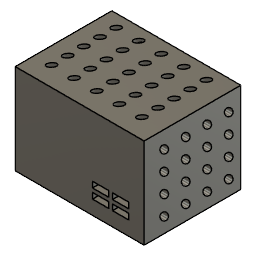
dronebox (Autodesk Fusion 360 design; units mm, degrees)
part number: 2026-05-27-13-25-45-977
Autodesk Fusion 360 part; units mm, degrees
sketch "Sketch12" plane through (0, 0, 0) normal (0, 0, 1) x (1, 0, 0)
  line L0 (50, 35) -> (-50, 35)
  line L1 (-50, 35) -> (-50, -35)
  line L2 (-50, -35) -> (50, -35)
  line L3 (50, -35) -> (50, 35)
  line L4 (50, 35) -> (-50, -35) construction
  line L5 (-50, 35) -> (50, -35) construction
  line L6 (-50, 35) -> (-50, 31)
  circle A0 centre (-20, 31) radius 1.6
  circle A1 centre (20, 31) radius 1.6
  circle A2 centre (-20, -31) radius 1.6
  circle A3 centre (20, -31) radius 1.6
  line L7 (42.5, -27.5) -> (42.5, 27.5)
  line L8 (42.5, 27.5) -> (-42.5, 27.5)
  line L9 (-42.5, 27.5) -> (-42.5, -27.5)
  line L10 (-42.5, -27.5) -> (42.5, -27.5)
  dimension "d61" = 100
  dimension "d62" = 70
  dimension "d63" = 4
  dimension "d64" = 30
  dimension "d65" = 3.2
  dimension "d66" = -7.5
  constraint horizontal L0
  constraint perpendicular L0 L1
  constraint parallel L0 L2
  constraint parallel L1 L3
  constraint coincident L4 origin
  constraint coincident L5 origin
  constraint perpendicular L0 L6
  measures "d61" distance of L1.end L2.end
  measures "d62" distance of L0.end L1.end
  measures "d63" distance of L0.end L6.end
  measures "d64" distance of L6.end A0.centre
  measures "d65" diameter of A0
extrude "Extrude12" add sketch "Sketch12" along normal blind 70 contours L0 L1 L2 L3 L6 | A0 | A1 | A2 | A3
extrude "Extrude13" cut sketch "Sketch12" along normal blind 15 contours A0 | A1 | A2 | A3
sketch "Sketch15" plane through (42.5, 0, 0) normal (-1, 0, 0) x (0, 0, 1)
  line L0 (0, 27.5) -> (0, -27.5)
  line L1 (0, -27.5) -> (70, -27.5)
  line L2 (70, -27.5) -> (70, 27.5)
  line L3 (70, 27.5) -> (0, 27.5)
sketch "Sketch16" plane through (-50, 0, 0) normal (-1, 0, 0) x (0, 0, 1)
  line L0 (0, 35) -> (0, -35)
  line L1 (0, -35) -> (70, -35)
  line L2 (70, -35) -> (70, 35)
  line L3 (70, 35) -> (0, 35)
  ellipse E0 centre (59.4117, -23.4278) end of major axis (56.6555, -26.4903) minor radius 2.5302
  line L4 (62.168, -20.3654) -> (56.6555, -26.4903) construction
  line L5 (57.5311, -21.7352) -> (61.2924, -25.1204) construction
  ellipse E1 centre (42.7451, -23.4278) end of major axis (39.9889, -26.4903) minor radius 2.5302
  ellipse E2 centre (26.0784, -23.4278) end of major axis (23.3222, -26.4903) minor radius 2.5302
  ellipse E3 centre (9.4117, -23.4278) end of major axis (6.6555, -26.4903) minor radius 2.5302
  ellipse E4 centre (59.4117, -8.4278) end of major axis (56.6555, -11.4903) minor radius 2.5302
  ellipse E5 centre (42.7451, -8.4278) end of major axis (39.9889, -11.4903) minor radius 2.5302
  ellipse E6 centre (26.0784, -8.4278) end of major axis (23.3222, -11.4903) minor radius 2.5302
  ellipse E7 centre (9.4117, -8.4278) end of major axis (6.6555, -11.4903) minor radius 2.5302
  ellipse E8 centre (59.4117, 6.5722) end of major axis (56.6555, 3.5097) minor radius 2.5302
  ellipse E9 centre (42.7451, 6.5722) end of major axis (39.9889, 3.5097) minor radius 2.5302
  ellipse E10 centre (26.0784, 6.5722) end of major axis (23.3222, 3.5097) minor radius 2.5302
  ellipse E11 centre (9.4117, 6.5722) end of major axis (6.6555, 3.5097) minor radius 2.5302
  ellipse E12 centre (59.4117, 21.5722) end of major axis (56.6555, 18.5097) minor radius 2.5302
  ellipse E13 centre (42.7451, 21.5722) end of major axis (39.9889, 18.5097) minor radius 2.5302
  ellipse E14 centre (26.0784, 21.5722) end of major axis (23.3222, 18.5097) minor radius 2.5302
  ellipse E15 centre (9.4117, 21.5722) end of major axis (6.6555, 18.5097) minor radius 2.5302
  dimension "d79" = -50
  dimension "d80" = 45
  constraint coincident E0 L4.start
  constraint coincident E0 L4.end
  constraint coincident E0 L5.start
  constraint coincident E0 L5.end
extrude "Extrude15" cut sketch "Sketch16" against normal blind 390 contours E0 | E1 | E2 | E3 | E4 | E5 | E6 | E7 | E8 | E9 | E10 | E11 | E12 | E13 | E14 | E15
sketch "Sketch17" plane through (0, 35, 0) normal (0, 1, 0) x (-1, 0, 0)
  line L0 (-50, 0) -> (50, 0)
  line L1 (50, 0) -> (50, 70)
  line L2 (50, 70) -> (-50, 70)
  line L3 (-50, 70) -> (-50, 0)
  ellipse E0 centre (36.9027, 9.7999) end of major axis (34.7589, 7.0437) minor radius 2.2086
  line L4 (39.0464, 12.5561) -> (34.7589, 7.0437) construction
  line L5 (35.1593, 11.1558) -> (38.646, 8.4439) construction
  ellipse E1 centre (19.4027, 9.7999) end of major axis (17.2589, 7.0437) minor radius 2.2086
  ellipse E2 centre (1.9027, 9.7999) end of major axis (-0.2411, 7.0437) minor radius 2.2086
  ellipse E3 centre (-15.5973, 9.7999) end of major axis (-17.7411, 7.0437) minor radius 2.2086
  ellipse E4 centre (-33.0973, 9.7999) end of major axis (-35.2411, 7.0437) minor radius 2.2086
  ellipse E5 centre (36.9027, 22.2999) end of major axis (34.7589, 19.5437) minor radius 2.2086
  ellipse E6 centre (19.4027, 22.2999) end of major axis (17.2589, 19.5437) minor radius 2.2086
  ellipse E7 centre (1.9027, 22.2999) end of major axis (-0.2411, 19.5437) minor radius 2.2086
  ellipse E8 centre (-15.5973, 22.2999) end of major axis (-17.7411, 19.5437) minor radius 2.2086
  ellipse E9 centre (-33.0973, 22.2999) end of major axis (-35.2411, 19.5437) minor radius 2.2086
  ellipse E10 centre (36.9027, 34.7999) end of major axis (34.7589, 32.0437) minor radius 2.2086
  ellipse E11 centre (19.4027, 34.7999) end of major axis (17.2589, 32.0437) minor radius 2.2086
  ellipse E12 centre (1.9027, 34.7999) end of major axis (-0.2411, 32.0437) minor radius 2.2086
  ellipse E13 centre (-15.5973, 34.7999) end of major axis (-17.7411, 32.0437) minor radius 2.2086
  ellipse E14 centre (-33.0973, 34.7999) end of major axis (-35.2411, 32.0437) minor radius 2.2086
  ellipse E15 centre (36.9027, 47.2999) end of major axis (34.7589, 44.5437) minor radius 2.2086
  ellipse E16 centre (19.4027, 47.2999) end of major axis (17.2589, 44.5437) minor radius 2.2086
  ellipse E17 centre (1.9027, 47.2999) end of major axis (-0.2411, 44.5437) minor radius 2.2086
  ellipse E18 centre (-15.5973, 47.2999) end of major axis (-17.7411, 44.5437) minor radius 2.2086
  ellipse E19 centre (-33.0973, 47.2999) end of major axis (-35.2411, 44.5437) minor radius 2.2086
  ellipse E20 centre (36.9027, 59.7999) end of major axis (34.7589, 57.0437) minor radius 2.2086
  ellipse E21 centre (19.4027, 59.7999) end of major axis (17.2589, 57.0437) minor radius 2.2086
  ellipse E22 centre (1.9027, 59.7999) end of major axis (-0.2411, 57.0437) minor radius 2.2086
  ellipse E23 centre (-15.5973, 59.7999) end of major axis (-17.7411, 57.0437) minor radius 2.2086
  ellipse E24 centre (-33.0973, 59.7999) end of major axis (-35.2411, 57.0437) minor radius 2.2086
  dimension "d85" = -70
  dimension "d86" = 50
  constraint coincident E0 L4.start
  constraint coincident E0 L4.end
  constraint coincident E0 L5.start
  constraint coincident E0 L5.end
extrude "Extrude16" cut sketch "Sketch17" against normal blind 85 contours E0 | E1 | E2 | E3 | E4 | E5 | E6 | E7 | E8 | E9 | E10 | E11 | E12 | E13 | E14 | E15 | E16 | E17 | E18 | E19 | E20 | E21 | E22 | E23 | E24
sketch "Sketch18" plane through (0, 0, 70) normal (0, 0, 1) x (1, 0, 0)
  line L0 (42.5, -27.5) -> (-42.5, -27.5)
  line L1 (-42.5, -27.5) -> (-42.5, 27.5)
  line L2 (-42.5, 27.5) -> (42.5, 27.5)
  line L3 (42.5, 27.5) -> (42.5, -27.5)
  line L4 (-50, 35) -> (-50, -35)
  line L5 (-50, -35) -> (50, -35)
  line L6 (50, -35) -> (50, 35)
  line L7 (50, 35) -> (-50, 35)
extrude "Extrude17" add sketch "Sketch18" along normal blind 5 contours L0 L1 L2 L3 | L4 L5 L6 L7
sketch "Sketch19" plane through (0, 0, 75) normal (0, 0, 1) x (1, 0, 0)
  line L0 (50, 35) -> (-50, 35)
  line L1 (-50, 35) -> (-50, -35)
  line L2 (-50, -35) -> (50, -35)
  line L3 (50, -35) -> (50, 35)
sketch "Sketch20" plane through (0, 0, 70) normal (0, 0, -1) x (-1, 0, 0)
  line L0 (-42.5, 27.5) -> (-42.5, -27.5)
  line L1 (-42.5, -27.5) -> (42.5, -27.5)
  line L2 (42.5, -27.5) -> (42.5, 27.5)
  line L3 (42.5, 27.5) -> (-42.5, 27.5)
sketch "Sketch21" plane through (0, 0, 75) normal (0, 0, 1) x (1, 0, 0)
  line L0 (50, 35) -> (-50, 35)
  line L1 (-50, 35) -> (-50, -35)
  line L2 (-50, -35) -> (50, -35)
  line L3 (50, -35) -> (50, 35)
  line L4 (38, -24) -> (10, -24)
  line L5 (10, -24) -> (10, -12)
  line L6 (10, -12) -> (38, -12)
  line L7 (38, -12) -> (38, -24)
  line L8 (24, -24) -> (24, -12)
  line L9 (38, -18) -> (10, -18)
  line L10 (25.5, -24) -> (25.5, -12)
  line L11 (22.5, -24) -> (22.5, -12)
  line L12 (38, -16.5) -> (10, -16.5)
  line L13 (38, -19.5) -> (10, -19.5)
  dimension "d91" = 1.5
  dimension "d92" = -1.5
  dimension "d93" = 1.5
  dimension "d94" = -1.5
  constraint horizontal L4
  constraint vertical L5
  constraint horizontal L6
  constraint vertical L7
  constraint midpoint L4 L8.start
  constraint midpoint L6 L8.end
  constraint midpoint L7 L9.start
  constraint midpoint L5 L9.end
extrude "Extrude18" cut sketch "Sketch21" against normal blind 44 contours L4 L5 L11 L13
extrude "Extrude19" cut sketch "Sketch21" against normal blind 22 contours L5 L6 L11 L12
extrude "Extrude20" cut sketch "Sketch21" against normal blind 17 contours L4 L7 L10 L13 | L6 L7 L10 L12
equation "d92 = -d91"
equation "d94 = -d93"
